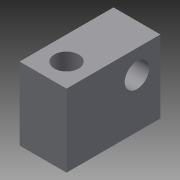
# Autodesk Inventor part: roller_joint_front
Saved by Autodesk Inventor 2015 (Build 190159000, 159)
## iProperties
Created: 2017-12-05
Part Number: roller_joint_front
Material: Generic
Document SubType Name: Modeling
Designer: Anshul
Density: 1 g/cm^3
Appearance: Default
Author: Anshul
Autodesk Inventor part; units mm, degrees
ref_plane "YZ Plane" through (0, 0, 0) normal (1, 0, 0) x (0, 1, 0)
ref_plane "XZ Plane" through (0, 0, 0) normal (0, 1, 0) x (-1, 0, 0)
ref_plane "XY Plane" through (0, 0, 0) normal (0, 0, 1) x (1, 0, 0)
sketch "Sketch1" plane through (0, 0, 0) normal (0, 1, 0) x (-1, 0, 0)
  line L0 (0, 0) -> (0, -5.5)
  line L1 (0, -5.5) -> (0, -15.5)
  circle A0 centre (0, -15.5) radius 2.6
  line L2 (0, -100) -> (0, -84.8)
  circle A1 centre (0, -84.8) radius 2.6
  line L3 (0, -50) -> (0, -26)
  line L4 (0, -26) -> (-5, -26)
  line L5 (0, -12.9) -> (0, -10.5)
  line L6 (0, -10.5) -> (-5, -10.5)
  line L7 (-5, -10.5) -> (-5, -26)
  line L8 (0, -10.5) -> (5, -10.5)
  line L9 (5, -10.5) -> (5, -26)
  line L10 (5, -26) -> (0, -26)
  line L11 (0, 0) -> (0, -12.9)
  line L12 (0, -18.1) -> (0, -100)
  line L13 (0, 0) -> (5, 0)
  line L14 (0, 0) -> (-5, 0)
  line L15 (0, 0) -> (0, 5)
  line L16 (0, 5) -> (0, 12.4)
  line L17 (0, 15) -> (0, 20)
  line L18 (0, 20) -> (-5, 20)
  line L19 (-5, 20) -> (-5, 0)
  line L20 (5, 0) -> (5, 20)
  line L21 (5, 20) -> (0, 20)
  circle A2 centre (0, 15) radius 2.6
  dimension "d15" = 5.2
  dimension "d0" = 100
  dimension "d1" = 5.5
  dimension "d2" = 10
  dimension "d3" = 5.2
  dimension "d4" = 15.2
  dimension "d5" = 5.2
  dimension "d6" = 24
  dimension "d7" = 5
  dimension "d8" = 5
  dimension "d9" = 5
  dimension "d10" = 5
  dimension "d11" = 5
  dimension "d12" = 5
  dimension "d13" = 10
  dimension "d14" = 5
  constraints: 44 end point, 10 point on line, 8 perpendicular, 3 coincident, 2 centre point, 2 horizontal, 2 point on circle, 2 vertical, 1 midpoint, 1 parallel, 1 vertical alignment, 2 other
  measures "d0" distance of L0.start L2.start
  measures "d1" distance of L0.start L0.end
  measures "d2" distance of L0.end L1.end
  measures "d3" diameter of A0
  measures "d4" distance of L2.start L2.end
  measures "d5" diameter of A1
  measures "d6" distance of L3.start L3.end
  measures "d7" distance of L3.end L4.end
  measures "d8" distance of A0.centre L5.end
  measures "d9" distance of L5.end L8.end
  measures "d10" distance of L0.start L13.end
  measures "d11" distance of L0.start L14.end
  measures "d12" distance of L0.start L15.end
  measures "d13" distance of L15.end L17.start
  measures "d14" distance of L17.start L17.end
extrude "Extrusion1" add sketch "Sketch1" along normal blind 15.5 contours L15 L16 A2 L17 L21 L20 L13 | L14 L19 L18 L17 A2 L16 L15
sketch "Sketch2" plane through (5, 0, 20) normal (1, 0, 0) x (0, 0, -1)
  line L0 (20, 15.5) -> (15, 15.5)
  line L1 (20, 15.5) -> (0, 15.5) projected
  line L2 (15, 15.5) -> (15, 10.5)
  circle A0 centre (15, 10.5) radius 2.6
  point P0 (20, 0)
  dimension "d18" = 5
  dimension "d19" = 5
  dimension "d20" = 5.2
  constraints: 4 end point, 1 centre point, 1 coincident, 1 perpendicular, 1 point on line
  measures "d18" distance of L0.start L0.end
  measures "d19" distance of L0.end L2.end
  measures "d20" diameter of A0
extrude "Extrusion2" cut sketch "Sketch2" against normal blind 15.5
body "Solid1"
